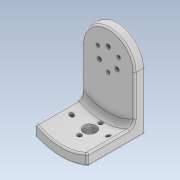
# Autodesk Inventor part: thigh_hip_connector
Saved by Autodesk Inventor 2020 (Build 240168000, 168)
## iProperties
Created: 2021-01-06
Part Number: thigh_hip_connector
Material: Generic
Document SubType Name: Modeling
Designer: DELL
Density: 1 g/cm^3
Appearance: Clear - Blue
Author: DELL
Autodesk Inventor part; units mm, degrees
ref_plane "YZ Plane" through (0, 0, 0) normal (1, 0, 0) x (0, 1, 0)
ref_plane "XZ Plane" through (0, 0, 0) normal (0, 1, 0) x (-1, 0, 0)
ref_plane "XY Plane" through (0, 0, 0) normal (0, 0, 1) x (1, 0, 0)
sketch "Sketch1" plane through (0, 0, 0) normal (0, 0, 1) x (1, 0, 0)
  circle A0 centre (0, 0) radius 25
  line L0 (-25, 0) -> (-25, -54.5436)
  line L1 (25, 0) -> (25, -54.5436)
  line L2 (9.9593, -5.75) -> (0, 0) construction
  circle A1 centre (8.4134, -4.8575) radius 2
  line L3 (0, 0) -> (9.9593, 5.75) construction
  line L4 (0, 0) -> (-9.9593, -5.75) construction
  circle A2 centre (-8.4134, -4.8575) radius 2
  circle A3 centre (0, 0) radius 9.715 construction
  circle A4 centre (0, 0) radius 11.5 construction
  circle A5 centre (0, 9.715) radius 2
  line L5 (0, 0) -> (-9.9593, 5.75) construction
  line L6 (11.5, 0) -> (-11.5, 0) construction
  circle A6 centre (-9.9593, 5.75) radius 2.75
  circle A7 centre (-9.9593, 5.75) radius 1.65
  line L7 (0, -48.5721) -> (0, 22.5) construction
  circle A8 centre (0, -11.5) radius 1.65
  circle A9 centre (0, -11.5) radius 2.75
  circle A10 centre (9.9593, 5.75) radius 2.75
  circle A11 centre (9.9593, 5.75) radius 1.65
  arc A12 (-25, -43.3013) -> (25, -43.3013) centre (0, 0) ccw
  arc A13 (-25, -54.5436) -> (25, -54.5436) centre (0, 0) ccw
  point P0 (0, 11.4686)
  point P1 (0, 11.4686)
  point P2 (11.5, 0)
  point P3 (-11.5, 0)
  dimension "d18" = 23
  dimension "d0" = 50
  dimension "d17" = 19.43
  dimension "d19" = 30
  dimension "d20" = 30
  dimension "d21" = 3.3
  dimension "d22" = 5.5
  dimension "d23" = 4
  dimension "d24" = 100
  dimension "d25" = 120
  constraints: 14 end point, 13 centre point, 10 coincident, 9 point on circle, 8 point on line, 6 equal radius, 3 vertical, 2 tangent, 16 other
  measures "d0" diameter of A0
  measures "d17" diameter of A3
  measures "d19" angle to the sketch x axis of L5
  measures "d20" angle to the sketch x axis of L4
  measures "d21" diameter of A11
  measures "d22" diameter of A10
  measures "d23" diameter of A5
  measures "d24" diameter of A12
  measures "d25" diameter of A13
extrude "Extrusion1" add sketch "Sketch1" along normal blind 10 contours A0 | L1 A12 L0 A0 | L1 A13 L0 A12 | A1 | A2 | A5 | A6 | A9 | A10
extrude "Extrusion2" cut sketch "Sketch1" along normal blind 5 contours A6 | A9 | A10 | A11
extrude "Extrusion3" cut sketch "Sketch1" against normal blind 5 from surface at 10 contours A1 | A2 | A5
extrude "Extrusion4" add sketch "Sketch1" along normal blind 45 from surface at 10 contours L1 A13 L0 A12
fillet "Fillet1" radius 5 1 edges at (0, -50, 10)
fillet "Fillet2" radius 1.5 17 edges at (0, -60, 0) (0, -60, 55) (25, -54.5436, 27.5) (-25, -54.5436, 27.5) (-25, -27.2718, 0) (25, -27.2718, 0) (0, 25, 0) (-25, -18.7083, 10) (-25, -41.4222, 11.3171) (-25, -43.3013, 35) (25, -18.7083, 10) (25, -41.4222, 11.3171) (25, -43.3013, 35) (0, 25, 10) (0, -50, 55) (-25, -48.9224, 55) (25, -48.9224, 55)
sketch "Sketch2" plane through (0, 0, 0) normal (0, 1, 0) x (-1, 0, 0)
  circle A0 centre (0, 17.5) radius 2
  circle A1 centre (0, 37.5) radius 2
  circle A2 centre (0, 37.5) radius 1.25
  circle A3 centre (0, 17.5) radius 1.25
  line L0 (-25, 0) -> (-25, 55) construction
  line L1 (23.5, 0) -> (-23.5, 0) construction
  line L2 (23.5, 55) -> (-23.5, 55) construction
  line L3 (-25, 27.5) -> (25, 27.5) construction
  line L4 (25, 53.5) -> (25, 1.5) construction
  line L5 (-25, 53.5) -> (-25, 15) construction
  line L6 (0, 0) -> (0, 55) construction
  circle A4 centre (-17.5, 27.5) radius 1.25
  circle A5 centre (-17.5, 27.5) radius 2
  circle A6 centre (17.5, 27.5) radius 1.25
  circle A7 centre (17.5, 27.5) radius 2
  circle A8 centre (0, 27.5) radius 6
  circle A9 centre (0, 27.5) radius 25
  dimension "d30" = 4
  dimension "d31" = 2.5
  dimension "d32" = 20
  dimension "d33" = 35
  dimension "d40" = 12
  dimension "d41" = 50
  constraints: 10 centre point, 6 end point, 6 equal radius, 5 coincident, 5 point on line, 4 midpoint, 2 symmetric about line, 1 collinear, 1 vertical
  measures "d30" diameter of A1
  measures "d31" diameter of A2
  measures "d32" distance of A1.centre A0.centre
  measures "d33" distance of A6.centre A4.centre
  measures "d40" diameter of A8
  measures "d41" diameter of A9
extrude "Extrusion5" cut sketch "Sketch2" against normal through all contours A2 | A3 | A4 | A6 | A8
extrude "Extrusion6" cut sketch "Sketch2" against normal blind 54 contours A0 | A1 | A2 | A3
extrude "Extrusion7" cut sketch "Sketch2" against normal up to surface (54 mm away) contours A4 | A5 | A6 | A7
body "Solid1"
